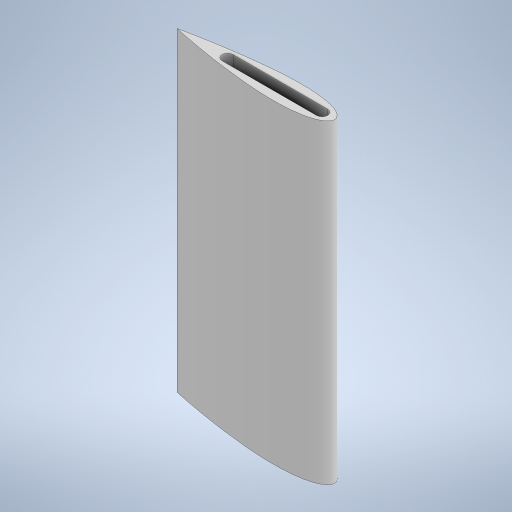
# Autodesk Inventor part: 0018
Saved by Autodesk Inventor 2023 (Build 270158000, 158)
## iProperties
Created: 2023-03-15
Part Number: 0018
Material: 一般
Document SubType Name: Modeling
Designer: USER
Density: 1 g/cm^3
Appearance: 預設
Author: USER
Autodesk Inventor part; units mm, degrees
ref_plane "YZ Plane" through (0, 0, 0) normal (1, 0, 0) x (0, 1, 0)
ref_plane "XZ Plane" through (0, 0, 0) normal (0, 1, 0) x (-1, 0, 0)
ref_plane "XY Plane" through (0, 0, 0) normal (0, 0, 1) x (1, 0, 0)
sketch "草圖1" plane through (0, 0, 0) normal (0, 1, 0) x (-1, 0, 0)
  spline S0 degree 5 poles (50, 0) (50, 0.0052) (49.9498, 0.0151) (49.7123, 0.0367) (49.6921, 0.1068) (49.0319, 0.1724) (48.7365, 0.3003) (47.8995, 0.4274) (47.1927, 0.6031) (46.1756, 0.7892) (45.1283, 1.0041) (43.9007, 1.2325) (42.5862, 1.4775) (41.1478, 1.7326) (39.6175, 1.9963) (37.9931, 2.2641) (36.2905, 2.5333) (34.5174, 2.8) (32.6859, 3.0609) (30.8071, 3.3124) (28.8923, 3.5503) (26.9536, 3.7713) (25.0027, 3.9706) (23.0517, 4.1449) (21.1126, 4.2895) (19.1973, 4.4009) (17.3176, 4.4752) (15.4849, 4.5095) (13.7106, 4.5008) (12.0056, 4.4473) (10.3801, 4.3477) (8.8443, 4.2017) (7.4073, 4.0099) (6.0778, 3.7736) (4.8637, 3.4949) (3.7715, 3.1768) (2.8072, 2.8219) (1.9747, 2.4335) (1.2774, 2.0124) (0.7179, 1.5601) (0.3031, 1.0726) (0.0436, 0.5525) (-0.042, 0) (0.0436, -0.5525) (0.3031, -1.0726) (0.7179, -1.5601) (1.2774, -2.0124) (1.9747, -2.4335) (2.8072, -2.8219) (3.7715, -3.1768) (4.8637, -3.4949) (6.0778, -3.7736) (7.4073, -4.0099) (8.8443, -4.2017) (10.3801, -4.3477) (12.0056, -4.4473) (13.7106, -4.5008) (15.4849, -4.5095) (17.3176, -4.4752) (19.1973, -4.4009) (21.1126, -4.2895) (23.0517, -4.1449) (25.0027, -3.9706) (26.9536, -3.7713) (28.8923, -3.5503) (30.8071, -3.3124) (32.6859, -3.0609) (34.5174, -2.8) (36.2905, -2.5333) (37.9931, -2.2641) (39.6175, -1.9963) (41.1478, -1.7326) (42.5862, -1.4775) (43.9007, -1.2325) (45.1283, -1.0041) (46.1756, -0.7892) (47.1927, -0.6031) (47.8995, -0.4274) (48.7365, -0.3003) (49.0319, -0.1724) (49.6921, -0.1068) (49.7123, -0.0367) (49.9498, -0.0151) (50, -0.0052) (50, 0) knots 0 0 0 0 0 0 0.005529 0.010356 0.017072 0.025226 0.03452 0.044785 0.055898 0.06776 0.080289 0.09341 0.107057 0.121168 0.135683 0.150547 0.165705 0.181105 0.196695 0.212424 0.228242 0.2441 0.259949 0.275739 0.291423 0.306953 0.322281 0.33736 0.352143 0.366584 0.380637 0.394255 0.407393 0.420006 0.43205 0.443487 0.454287 0.464441 0.473978 0.482987 0.491602 0.5 0.508398 0.517013 0.526022 0.535559 0.545713 0.556513 0.56795 0.579994 0.592607 0.605745 0.619363 0.633416 0.647857 0.66264 0.677719 0.693047 0.708577 0.724261 0.740051 0.7559 0.771758 0.787576 0.803305 0.818895 0.834295 0.849453 0.864317 0.878832 0.892943 0.90659 0.919711 0.93224 0.944102 0.955215 0.96548 0.974774 0.982928 0.989644 0.994471 1 1 1 1 1 1
  point P0 (0, 0)
  point P1 (49.6922, 0.0669)
  point P2 (49.3093, 0.1492)
  point P3 (48.7764, 0.2626)
  point P4 (48.097, 0.4049)
  point P5 (47.2751, 0.5738)
  point P6 (46.316, 0.7666)
  point P7 (45.2254, 0.9803)
  point P8 (44.0102, 1.2119)
  point P9 (42.6776, 1.4579)
  point P10 (41.2362, 1.7151)
  point P11 (39.6947, 1.9804)
  point P12 (38.0624, 2.25)
  point P13 (36.3498, 2.5208)
  point P14 (34.5671, 2.7891)
  point P15 (32.7254, 3.0514)
  point P16 (30.8361, 3.3041)
  point P17 (28.9109, 3.5431)
  point P18 (26.9615, 3.7647)
  point P19 (25, 3.9646)
  point P20 (23.0385, 4.1388)
  point P21 (21.0892, 4.2831)
  point P22 (19.1639, 4.3937)
  point P23 (17.2746, 4.4668)
  point P24 (15.4329, 4.4992)
  point P25 (13.6503, 4.4881)
  point P26 (11.9376, 4.4316)
  point P27 (10.3054, 4.3284)
  point P28 (8.7638, 4.1781)
  point P29 (7.3224, 3.9812)
  point P30 (5.9898, 3.739)
  point P31 (4.7746, 3.4537)
  point P32 (3.684, 3.1279)
  point P33 (2.7249, 2.765)
  point P34 (1.903, 2.3685)
  point P35 (1.2236, 1.942)
  point P36 (0.6907, 1.4891)
  point P37 (0.3078, 1.0128)
  point P38 (0.0771, 0.5158)
  point P39 (0, 0)
  point P40 (0.0771, -0.5158)
  point P41 (0.3078, -1.0128)
  point P42 (0.6907, -1.4891)
  point P43 (1.2236, -1.942)
  point P44 (1.903, -2.3685)
  point P45 (2.7249, -2.765)
  point P46 (3.684, -3.1279)
  point P47 (4.7746, -3.4537)
  point P48 (5.9898, -3.739)
  point P49 (7.3224, -3.9812)
  point P50 (8.7638, -4.1781)
  point P51 (10.3054, -4.3284)
  point P52 (11.9376, -4.4316)
  point P53 (13.6503, -4.4881)
  point P54 (15.4329, -4.4992)
  point P55 (17.2746, -4.4668)
  point P56 (19.1639, -4.3937)
  point P57 (21.0892, -4.2831)
  point P58 (23.0385, -4.1388)
  point P59 (25, -3.9646)
  point P60 (26.9615, -3.7647)
  point P61 (28.9109, -3.5431)
  point P62 (30.8361, -3.3041)
  point P63 (32.7254, -3.0514)
  point P64 (34.5671, -2.7891)
  point P65 (36.3498, -2.5208)
  point P66 (38.0624, -2.25)
  point P67 (39.6947, -1.9804)
  point P68 (41.2362, -1.7151)
  point P69 (42.6776, -1.4579)
  point P70 (44.0102, -1.2119)
  point P71 (45.2254, -0.9803)
  point P72 (46.316, -0.7666)
  point P73 (47.2751, -0.5738)
  point P74 (48.097, -0.4049)
  point P75 (48.7764, -0.2626)
  point P76 (49.3093, -0.1492)
  point P77 (49.6922, -0.0669)
  point P78 (49.923, -0.0168)
  constraints: 80 other
extrude "擠出2" add sketch "草圖1" along normal blind 100
sketch "草圖2" plane through (0, 100, 0) normal (0, 1, 0) x (1, 0, 0)
  line L0 (-4, 0) -> (-34, 0) construction
  line L1 (-4, 1.75) -> (-34, 1.75)
  line L2 (-34, -1.75) -> (-4, -1.75)
  arc A0 (-4, -1.75) -> (-4, 1.75) centre (-4, 0) ccw
  arc A1 (-34, 1.75) -> (-34, -1.75) centre (-34, 0) ccw
  point P0 (0, 0)
  point P1 (-19, 0)
  dimension "d4" = 3.5
  dimension "d5" = 4
  dimension "d6" = 30
  dimension "d7" = 19
  constraints: 8 end point, 4 point on circle, 4 tangent, 2 centre point, 1 horizontal, 1 midpoint, 1 parallel
  measures "d4" distance between parallel lines of L1 L2
  measures "d5" distance of point (0, 0) L0.start
  measures "d6" distance of L0.end L0.start
  measures "d7" distance of point (0, 0) point (-19, 0)
extrude "擠出3" cut sketch "草圖2" against normal through all
